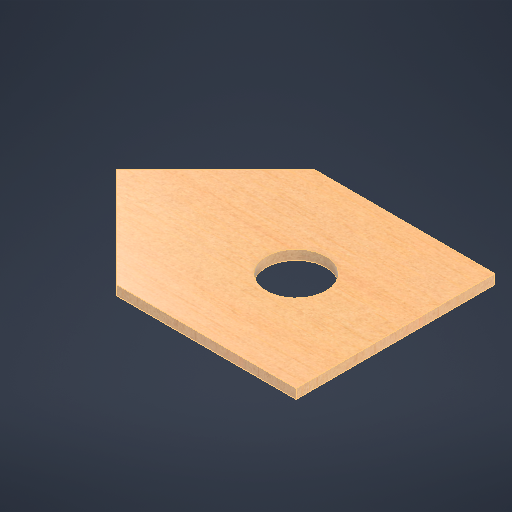
# Autodesk Inventor part: front wall
Saved by Autodesk Inventor 2026.2 (Build 302298000, 298)
## iProperties
Created: 2026-01-17
Part Number: front wall
Material: Pine
Document SubType Name: Modeling
Designer: User
Density: 0.570257 g/cm^3
Appearance: Yellow Pine - Solid Natural Low Gloss
Author: User
Autodesk Inventor part; units mm, degrees
ref_plane "YZ Plane" through (0, 0, 0) normal (1, 0, 0) x (0, 1, 0)
ref_plane "XZ Plane" through (0, 0, 0) normal (0, 1, 0) x (-1, 0, 0)
ref_plane "XY Plane" through (0, 0, 0) normal (0, 0, 1) x (1, 0, 0)
sketch "Sketch1" plane through (0, 0, 0) normal (0, 1, 0) x (-1, 0, 0)
  line L0 (0, 0) -> (180, 0)
  line L1 (180, 0) -> (180, -199.1625)
  line L2 (180, -199.1625) -> (0, -199.1625)
  line L3 (0, -199.1625) -> (0, 0)
  line L4 (180, 0) -> (279.5813, -99.5812)
  line L5 (279.5813, -99.5812) -> (180, -199.1625)
  circle A0 centre (99.5813, -99.5813) radius 30
  dimension "d0" = 199.1625
  dimension "d1" = 180
  dimension "d2" = 135
  dimension "d3" = 60
  dimension "d4" = 99.5812
  dimension "d5" = 99.5812
  constraints: 12 end point, 2 parallel, 2 perpendicular, 1 centre point, 1 horizontal
  measures "d0" distance of L2.end L0.start
  measures "d1" distance of L0.start L0.end
  measures "d2" angle of L1 L5
  measures "d3" diameter of A0
  measures "d4" distance from line of L3 A0.centre
  measures "d5" distance from line of L0 A0.centre
extrude "Extrusion1" add sketch "Sketch1" along normal blind 9.5813
ref_plane "Work Plane1" through (-180, 0, -99.5812) normal (0, 0, 1) x (1, 0, 0)
equation "\"d5\" = 0.5 * d0"
body "Solid1"
